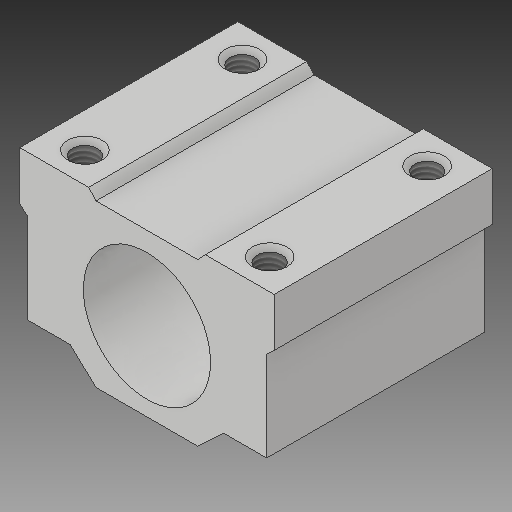
# Autodesk Inventor part: PilowBlockFechado
Saved by Autodesk Inventor 2018 (Build 220112000, 112)
## iProperties
Created: 2018-07-23
Part Number: PilowBlockFechado
Material: Genérico
Document SubType Name: Modeling
Designer: Usuario
Density: 1 g/cm^3
Appearance: Padrão
Mass: 23.3153 g
Surface Area: 97.1814 cm^2
Volume: 23.3153 cm^3
Author: Usuario
Autodesk Inventor part; units mm, degrees
ref_plane "YZ Plane" through (0, 0, 0) normal (1, 0, 0) x (0, 1, 0)
ref_plane "XZ Plane" through (0, 0, 0) normal (0, 1, 0) x (-1, 0, 0)
ref_plane "XY Plane" through (0, 0, 0) normal (0, 0, 1) x (1, 0, 0)
sketch "Esboço1" plane through (0, 0, 0) normal (0, 0, 1) x (1, 0, 0)
  circle A0 centre (5.38, 3.8406) radius 10.5
  line L0 (26.38, 18.8406) -> (26.38, 10.8406)
  line L1 (-15.62, 10.8406) -> (-15.62, 18.8406)
  line L2 (5.38, 32.1996) -> (5.38, -39.9391) construction
  line L3 (-9.87, 36.7798) -> (-9.87, -36.1222) construction
  line L4 (20.63, 36.7798) -> (20.63, -36.1222) construction
  line L5 (-15.62, 10.8406) -> (-14.3815, 9.6884)
  line L6 (-14.3815, 9.6884) -> (-14.3815, -5.1594)
  line L7 (26.38, 10.8406) -> (25.1416, 9.6884)
  line L8 (25.1416, 9.6884) -> (25.1416, -5.1594)
  line L9 (-7.3177, -5.1594) -> (-1.6608, -5.1594) construction
  line L10 (-7.3177, -5.1594) -> (-3.0182, -9.1594)
  line L11 (18.0777, -5.1594) -> (13.7782, -9.1594)
  line L12 (13.7782, -9.1594) -> (-3.0182, -9.1594)
  line L13 (-4.2504, 18.8406) -> (-3.0182, 17.516)
  line L14 (-3.0182, 17.516) -> (5.38, 17.516)
  line L15 (15.0105, 18.8406) -> (13.7782, 17.516)
  line L16 (13.7782, 17.516) -> (5.38, 17.516)
  line L17 (-15.62, 18.8406) -> (-4.2504, 18.8406)
  line L18 (15.0105, 18.8406) -> (26.38, 18.8406)
  line L19 (-14.3815, -5.1594) -> (-7.3177, -5.1594)
  line L20 (18.0777, -5.1594) -> (25.1416, -5.1594)
  dimension "d15" = 21
  dimension "d16" = 42
  dimension "d19" = 21
  dimension "d21" = 15.25
  dimension "d22" = 15.25
  dimension "d31" = 8
  constraints: 42 end point, 6 symmetric about line, 4 perpendicular, 4 vertical, 3 horizontal, 2 parallel, 1 centre point, 1 point on line
  measures "d15" diameter of A0
  measures "d16" distance of L1.end L0.start
  measures "d19" distance from line of L1 A0.centre
  measures "d21" distance between parallel lines of L3 L2
  measures "d22" distance between parallel lines of L2 L4
  measures "d31" distance of L1.start L1.end
extrude "Extrusão1" add sketch "Esboço1" against normal blind 36
sketch "Esboço2" plane through (15.0105, 18.8406, 0) normal (0, 1, 0) x (1, 0, 0)
  line L0 (15.0078, 18) -> (-43.7874, 18) construction
  line L1 (14.2178, 31) -> (-41.7561, 31) construction
  line L2 (14.2178, 5) -> (-36.0007, 5) construction
  line L3 (5.6195, 46.9459) -> (5.6195, -11.9622) construction
  line L4 (-24.8805, 46.9459) -> (-24.8805, -14.332) construction
  line L5 (-9.6305, -11.9622) -> (-9.6305, 51.9034) construction
  circle A0 centre (5.6195, 31) radius 2 construction
  circle A1 centre (5.6195, 5) radius 2 construction
  circle A2 centre (-24.8805, 31) radius 2 construction
  circle A3 centre (-24.8805, 5) radius 2 construction
  point P0 (-15.0105, 0)
  dimension "d36" = 13
  dimension "d37" = 13
  dimension "d38" = 15.25
  dimension "d39" = 15.25
  dimension "d40" = 4
  dimension "d41" = 4
  dimension "d42" = 4
  dimension "d43" = 4
  constraints: 12 end point, 8 point on line, 4 centre point, 4 horizontal, 4 vertical, 1 other
  measures "d36" distance between parallel lines of L0 L1
  measures "d37" distance between parallel lines of L0 L2
  measures "d38" distance between parallel lines of L5 L3
  measures "d39" distance between parallel lines of L4 L5
  measures "d40" diameter of A0
  measures "d41" diameter of A1
  measures "d42" diameter of A2
  measures "d43" diameter of A3
hole "Furo1" at (20.63, 18.8406, -31) at (20.63, 18.8406, -5) at (-9.87, 18.8406, -5) at (-9.87, 18.8406, -31) direction (0, -1, 0) diameter 4.134 end through all countersink diameter 5.7 countersink angle 90 thread size "M5x0.8" class "6H" standard "ANSI Metric M Profile"
equation "\"d22\" = d21"
equation "\"d37\" = d36"
equation "\"d39\" = d38"
